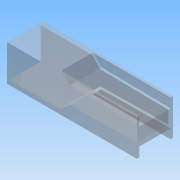
# Autodesk Inventor part: Cuvette
Saved by Autodesk Inventor 2016 (Build 200138000, 138)
## iProperties
Created: 2014-12-28
Part Number: Cuvette
Material: Polycarbonate, Clear
Document SubType Name: Modeling
Designer: Openlab
Density: 1.2 g/cm^3
Appearance: Polycarbonate - Clear
Mass: 15.3281 g
Surface Area: 25.625 cm^2
Volume: 7.03125 cm^3
Author: Openlab
Autodesk Inventor part; units mm, degrees
ref_plane "YZ Plane" through (0, 0, 0) normal (1, 0, 0) x (0, 1, 0)
ref_plane "XZ Plane" through (0, 0, 0) normal (0, 1, 0) x (-1, 0, 0)
ref_plane "XY Plane" through (0, 0, 0) normal (0, 0, 1) x (1, 0, 0)
sketch "Sketch1" plane through (0, 0, 0) normal (0, 1, 0) x (-1, 0, 0)
  line L0 (45, 0) -> (0, 0)
  line L1 (0, 0) -> (0, -12.5)
  line L2 (0, -12.5) -> (45, -12.5)
  line L3 (45, -12.5) -> (45, 0)
  dimension "d0" = 45
  dimension "d1" = 12.5
  constraints: 8 end point, 2 parallel, 1 coincident, 1 horizontal, 1 perpendicular
  measures "d0" distance of L2.end L1.end
  measures "d1" distance of L1.end L0.end
extrude "Extrusion1" add sketch "Sketch1" along normal blind 0.8
sketch "Sketch3" plane through (0, 0, 0) normal (0, -1, 0) x (1, 0, 0)
  line L0 (-45, 0) -> (-27, 0)
  line L1 (-27, 0) -> (-24, -2.9)
  line L2 (-24, -2.9) -> (0, -3.25)
  line L3 (0, 0) -> (0, -12.5) projected
  line L4 (0, -9.25) -> (-24, -9.6)
  line L5 (-24, -9.6) -> (-27, -12.5)
  line L6 (0, -12.5) -> (-45, -12.5) projected
  line L7 (-45, -12.5) -> (-27, -12.5)
  line L8 (0, 0) -> (0, -12.5) projected
  line L9 (-28.7719, -3.1178) -> (-25.8887, -3.1178) construction
  line L10 (-28.7189, -9.8202) -> (-22.671, -9.5806) construction
  line L11 (-45, 0) -> (0, 0) construction
  line L12 (0, -3.25) -> (0, -9.25)
  line L13 (-45, -12.5) -> (-45, 0) projected
  line L14 (-45, 0) -> (-45, -0.8)
  line L15 (-45, -0.8) -> (-27.3235, -0.8)
  line L16 (-27.3235, -0.8) -> (-24.3283, -3.6953)
  line L17 (-24.3283, -3.6953) -> (-0.8, -4.0384)
  line L18 (-0.8, -4.0384) -> (-0.8, -8.4616)
  line L19 (-0.8, -8.4616) -> (-24.3283, -8.8047)
  line L20 (-24.3283, -8.8047) -> (-27.3235, -11.7)
  line L21 (-27.3235, -11.7) -> (-45, -11.7)
  line L22 (-45, -12.5) -> (-45, -11.7)
  dimension "d6" = 18
  dimension "d7" = 6.7
  dimension "d9" = 2.9
  dimension "d10" = 6
  dimension "d12" = 24
  dimension "d13" = 3.25
  dimension "d14" = 0.8
  dimension "d15" = 0.8
  dimension "d16" = 0.8
  dimension "d17" = 0.8
  dimension "d18" = 0.8
  dimension "d19" = 0.8
  dimension "d20" = 0.8
  constraints: 36 end point, 6 point on line, 3 horizontal, 3 perpendicular, 2 collinear, 2 parallel, 2 vertical alignment
  measures "d6" distance of L0.start L0.end
  measures "d7" distance of L4.end L1.end
  measures "d9" distance from line of L0 L1.end
  measures "d10" distance of L4.start L2.end
  measures "d12" distance from line of L3 L1.end
  measures "d13" distance from line of L0 L2.end
  measures "d14" distance of L0.start L14.end
  measures "d15" distance between parallel lines of L1 L16
  measures "d16" distance between parallel lines of L2 L17
  measures "d17" distance between parallel lines of L12 L18
  measures "d18" distance of L6.end L21.end
  measures "d19" distance between parallel lines of L20 L5
  measures "d20" distance between parallel lines of L19 L4
extrude "Extrusion2" add sketch "Sketch3" along normal blind 10.9 contours L0 L1 L2 L3 L4 L5 L6 L13 L21 L20 L19 L18 L17 L16 L15
sketch "Sketch4" plane through (0, -10.9, 0) normal (0, -1, 0) x (1, 0, 0)
  line L0 (0, 0) -> (0, -12.5) projected
  line L1 (-45, 0) -> (0, 0)
  line L2 (0, 0) -> (0, -12.5)
  line L3 (0, -12.5) -> (-45, -12.5)
  line L4 (-45, -12.5) -> (-45, 0)
  constraints: 8 end point, 2 parallel, 1 horizontal, 1 perpendicular
extrude "Extrusion3" add sketch "Sketch4" along normal blind 0.8
body "Solid1"
